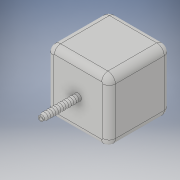
# Autodesk Inventor part: Square-Circle-Adapter V2D2-OUT
Saved by Autodesk Inventor 2017 (Build 210142000, 142)
## iProperties
Created: 2017-12-22
Part Number: Square-Circle-Adapter V2D2-OUT
Material: Generic
Document SubType Name: Modeling
Designer: Tripl_000
Density: 1 g/cm^3
Appearance: Default
Author: Tripl_000
Autodesk Inventor part; units mm, degrees
ref_plane "YZ Plane" through (0, 0, 0) normal (1, 0, 0) x (0, 1, 0)
ref_plane "XZ Plane" through (0, 0, 0) normal (0, 1, 0) x (-1, 0, 0)
ref_plane "XY Plane" through (0, 0, 0) normal (0, 0, 1) x (1, 0, 0)
sketch "Sketch1" plane through (0, 0, 0) normal (0, 0, 1) x (1, 0, 0)
  line L0 (-12.7, 12.7) -> (12.7, 12.7)
  line L1 (12.7, 12.7) -> (12.7, -12.7)
  line L2 (12.7, -12.7) -> (-12.7, -12.7)
  line L3 (-12.7, -12.7) -> (-12.7, 12.7)
  line L4 (-12.7, 12.7) -> (12.7, -12.7) construction
  line L5 (12.7, 12.7) -> (-12.7, -12.7) construction
  point P0 (0, 0)
  dimension "d0" = 25.4
  dimension "d1" = 25.4
  constraints: 12 end point, 2 midpoint, 2 parallel, 1 horizontal, 1 perpendicular
  measures "d0" distance of L2.end L0.start
  measures "d1" distance of L0.start L0.end
extrude "Extrusion1" add sketch "Sketch1" along normal blind 15
sketch "Sketch2" plane through (0, 0, 15) normal (0, 0, 1) x (1, 0, 0)
  line L0 (-6.604, 6.604) -> (6.604, 6.604)
  line L1 (6.604, 6.604) -> (6.604, -6.604)
  line L2 (6.604, -6.604) -> (-6.604, -6.604)
  line L3 (-6.604, -6.604) -> (-6.604, 6.604)
  line L4 (-6.604, 6.604) -> (6.604, -6.604) construction
  line L5 (6.604, 6.604) -> (-6.604, -6.604) construction
  point P0 (0, 0)
  dimension "d4" = 13.208
  dimension "d5" = 13.208
  constraints: 12 end point, 2 midpoint, 2 parallel, 1 horizontal, 1 perpendicular
  measures "d4" distance of L0.end L1.end
  measures "d5" distance of L0.start L0.end
extrude "Extrusion2" cut sketch "Sketch2" against normal through all
sketch "Sketch5" plane through (0, 0, 15) normal (0, 0, 1) x (1, 0, 0)
  line L0 (12.7, 12.7) -> (-12.7, 12.7) projected
  line L1 (12.7, 12.7) -> (12.7, -12.7) projected
  line L2 (-12.7, 12.7) -> (12.7, 12.7)
  line L3 (12.7, 12.7) -> (12.7, -12.7)
  line L4 (12.7, -12.7) -> (-12.7, -12.7)
  line L5 (-12.7, -12.7) -> (-12.7, 12.7)
  point P0 (0, 0)
  constraints: 8 end point, 2 parallel, 1 horizontal, 1 perpendicular
extrude "Extrusion5" add sketch "Sketch5" along normal blind 10
sketch "Sketch8" plane through (0, 0, 25) normal (0, 0, 1) x (1, 0, 0)
  circle A0 centre (0, 0) radius 0.762
  dimension "d44" = 1.524
  constraints: 1 centre point, 1 coincident
  measures "d44" diameter of A0
extrude "Extrusion7" add sketch "Sketch8" along normal blind 15.24
sketch "Sketch9" plane through (0, 0, 25) normal (0, 0, 1) x (1, 0, 0)
  circle A0 centre (0, 0) radius 1.016
  dimension "d47" = 2.032
  constraints: 1 centre point, 1 coincident
  measures "d47" diameter of A0
extrude "Extrusion8" add sketch "Sketch9" along normal up to surface (15.24 mm away)
ref_plane "Work Plane3" through (0, -12.7, 0) normal (1, 0, 0) x (0, 0, -1)
sketch "Sketch10" plane through (0, -12.7, 0) normal (1, 0, 0) x (0, 0, -1)
  line L0 (21.7384, 12.7) -> (-63.7893, 12.7)
  line L1 (-25, 11.684) -> (-25, 13.716) projected
  line L2 (-25, 13.716) -> (-25, 14.097)
  line L3 (-25, 0) -> (-25, 25.4) projected
  line L4 (-25, 14.097) -> (-26.0468, 13.716)
  line L5 (-25, 13.716) -> (-40.24, 13.716) projected
  line L6 (-26.0468, 13.716) -> (-26.0468, 14.097)
  line L7 (-26.0468, 14.097) -> (-27.0936, 13.716)
  line L8 (-27.0936, 13.716) -> (-27.0936, 14.097)
  line L9 (-27.0936, 14.097) -> (-28.1404, 13.716)
  line L10 (-28.1404, 13.716) -> (-28.1404, 14.097)
  line L11 (-28.1404, 14.097) -> (-29.1872, 13.716)
  line L12 (-29.1872, 13.716) -> (-29.1872, 14.097)
  line L13 (-29.1872, 14.097) -> (-30.2339, 13.716)
  line L14 (-30.2339, 13.716) -> (-30.2339, 14.097)
  line L15 (-30.2339, 14.097) -> (-31.2807, 13.716)
  line L16 (-31.2807, 13.716) -> (-31.2807, 14.097)
  line L17 (-31.2807, 14.097) -> (-32.3275, 13.716)
  line L18 (-32.3275, 13.716) -> (-32.3275, 14.097)
  line L19 (-32.3275, 14.097) -> (-33.3743, 13.716)
  line L20 (-33.3743, 13.716) -> (-33.3743, 14.097)
  line L21 (-33.3743, 14.097) -> (-34.4211, 13.716)
  line L22 (-34.4211, 13.716) -> (-34.4211, 14.097)
  line L23 (-34.4211, 14.097) -> (-35.4679, 13.716)
  line L24 (-35.4679, 13.716) -> (-35.4679, 14.097)
  line L25 (-35.4679, 14.097) -> (-36.5147, 13.716)
  line L26 (-36.5147, 13.716) -> (-36.5147, 14.097)
  line L27 (-36.5147, 14.097) -> (-37.5615, 13.716)
  line L28 (-37.5615, 13.716) -> (-37.5615, 14.097)
  line L29 (-37.5615, 14.097) -> (-38.6083, 13.716)
  line L30 (-38.6083, 13.716) -> (-38.6083, 14.097)
  line L31 (-38.6083, 14.097) -> (-39.655, 13.716)
  line L32 (0, 0) -> (-25, 0) projected
  point P0 (0, 12.7)
  dimension "d51" = 0.381
  dimension "d52" = 70
  dimension "d87" = 12.7
  constraints: 58 end point, 13 vertical, 10 parallel, 1 horizontal, 1 point on line, 15 other
  measures "d51" distance of L1.end L2.end
  measures "d52" angle of L2 L4
  measures "d87" distance between parallel lines of L32 L0
revolve "Revolution3" add sketch "Sketch10" angle 360 about axis through (0, 0, -21.7384) along (0, 0, 1)
sketch "Sketch11" plane through (0, 0, 40.24) normal (0, 0, 1) x (1, 0, 0)
  circle A0 centre (0, 0) radius 0.635
  dimension "d79" = 1.27
  constraints: 1 centre point, 1 coincident
  measures "d79" diameter of A0
extrude "Extrusion9" cut sketch "Sketch11" against normal through all
sketch "Sketch12" plane through (0, -12.7, 0) normal (1, 0, 0) x (0, 0, -1)
  point P0 (0, 12.7)
fillet "Fillet13" radius 1.27 1 edges at (-0.635, 0, 15)
fillet "Fillet14" radius 2.54 4 edges at (-6.604, 6.604, 7.5) (6.604, 6.604, 7.5) (6.604, -6.604, 7.5) (-6.604, -6.604, 7.5)
fillet "Fillet15" radius 3.048 4 edges at (12.7, 12.7, 12.5) (-12.7, 12.7, 12.5) (12.7, -12.7, 12.5) (-12.7, -12.7, 12.5)
fillet "Fillet16" radius 5.207 8 edges at (-5.8601, -5.8601, 15) (-6.604, 0, 15) (-5.8601, 5.8601, 15) (0, 6.604, 15) (5.8601, 5.8601, 15) (6.604, 0, 15) (5.8601, -5.8601, 15) (0, -6.604, 15)
fillet "Fillet17" radius 2.54 16 edges at (11.8073, 11.8073, 0) (12.7, 0, 0) (11.8073, -11.8073, 0) (0, -12.7, 0) (-11.8073, -11.8073, 0) (-12.7, 0, 0) (-11.8073, 11.8073, 0) (0, 12.7, 0) (-11.8073, 11.8073, 25) (-12.7, 0, 25) (-11.8073, -11.8073, 25) (0, -12.7, 25) (11.8073, -11.8073, 25) (12.7, 0, 25) (11.8073, 11.8073, 25) (0, 12.7, 25)
body "Solid1"
